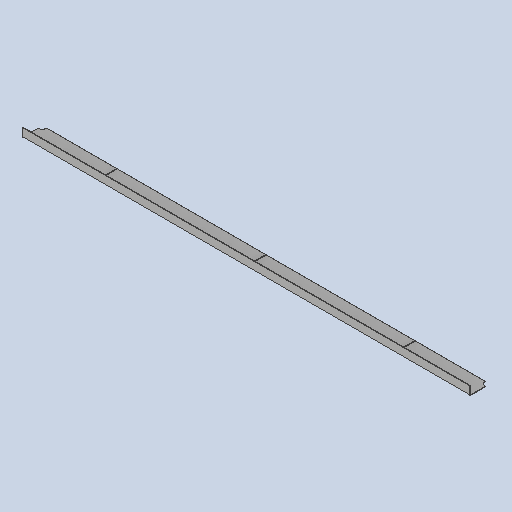
# Autodesk Inventor part: МОО 052 стрингер спина 21
Saved by Autodesk Inventor 2024.2 (Build 282272000, 272)
## iProperties
Created: 2024-04-28
Part Number: МОО 052 стрингер спина 21
Material: Stainless Steel
Document SubType Name: Sheet Metal
Designer: pokla
Density: 8 g/cm^3
Sheet Metal Rule: AISI304 2mm Die16
Appearance: Default
Flat Pattern Width: 9.3976 cm
Flat Pattern Length: 150 cm
Flat Pattern Area: 1409.64 cm^2
Sheet Metal Width: 93,976 mm
Sheet Metal Length: 1500,000 mm
Sheet Metal Area: 140964,031 mm^2
Author: admin
Autodesk Inventor part; units mm, degrees
ref_plane "YZ Plane" through (0, 0, 0) normal (1, 0, 0) x (0, 1, 0)
ref_plane "XZ Plane" through (0, 0, 0) normal (0, 1, 0) x (-1, 0, 0)
ref_plane "XY Plane" through (0, 0, 0) normal (0, 0, 1) x (1, 0, 0)
sketch "Sketch1" plane through (0, 0, 0) normal (0, 0, 1) x (1, 0, 0)
  line L0 (-750, 67.4521) -> (750, 67.4521)
  line L1 (750, 67.4521) -> (750, 0)
  line L2 (750, 0) -> (-750, 0)
  line L3 (-750, 0) -> (-750, 67.4521)
  point P0 (0, 0)
  point P1 (0, 0)
  dimension "d0" = 1500
  dimension "d1" = 67.4521
  measures "d0" distance of L1.end L2.end
  measures "d1" distance of L0.end L1.end
extrude "Plate1" add sketch "Sketch1" along normal blind 2
sketch "Sketch2" plane through (750, 2, 0) normal (0, -1, 0) x (1, 0, 0)
  line L0 (-1500, 0) -> (0, 0)
  line L1 (0, 0) -> (0, 30)
  line L2 (0, 30) -> (-1500, 30)
  line L3 (-1500, 30) -> (-1500, 0)
  constraints: 6 end point, 1 horizontal, 1 perpendicular, 1 vertical
edge flange "Flange1" height 30 angle 90 thickness 2 bend radius 2 thickness toward (0, -1, 0) relief tear relief width 2 relief depth 1 edges at (0, 0, 2) wall of the first edge with corners at (-750, 2, 0) (750, 2, 0) (750, 2, 30) (-750, 2, 30)
bend "Bend1"
corner "Corner1"
sketch "Sketch5" plane through (0, 0, 0) normal (0, 0, -1) x (-1, 0, 0)
  line L0 (750, 67.4521) -> (-750, 67.4521) projected
  line L1 (499, 67.4521) -> (499, 29)
  line L2 (499, 29) -> (501, 29)
  line L3 (501, 29) -> (501, 67.4521)
  line L4 (750, 0) -> (-750, 0) projected
  point P0 (0, 0)
  point P1 (500, 29)
  dimension "d18" = 2
  dimension "d20" = 29
  dimension "d27" = 250
  constraints: 6 end point, 2 perpendicular, 2 point on line, 1 midpoint, 1 vertical
  measures "d18" distance between parallel lines of L3 L1
  measures "d20" distance between parallel lines of L4 L2
  measures "d27" horizontal distance of point (500, 29) L0.start
extrude "Extrusion1" cut sketch "Sketch5" against normal through all
pattern_linear "Rectangular Pattern1" count 3 spacing 500 along (1, 0, 0) of "Extrusion1"
sketch "Sketch6" plane through (0, 0, 0) normal (0, 0, -1) x (-1, 0, 0)
  line L0 (-750, 67.4521) -> (-750, 4) projected
  circle A0 centre (-750, 67.4521) radius 15
  line L1 (-750, 67.4521) -> (-501, 67.4521) projected
  point P0 (0, 0)
  point P1 (-735, 67.4521)
  point P2 (-750, 52.4521)
  dimension "d24" = 30
  constraints: 1 centre point
  measures "d24" diameter of A0
extrude "Extrusion2" cut sketch "Sketch6" against normal through all contours L1 A0 L0 picked at (-740.1254, 66.3395)
mirror "Mirror1" about plane through (0, 0, 0) normal (1, 0, 0) of "Extrusion2"
equation "\"d1\" = Стрингер_2"
equation "\"d18\" = Thickness"
equation "\"d2\" = Thickness"
equation "\"d3\" = BendReliefWidth"
equation "\"d4\" = BendReliefDepth"
equation "\"d5\" = MinimumRemnant"
equation "\"d6\" = TransitionRadius"
equation "\"d9\" = BendRadius"
equation "\"d10\" = CornerReliefSize"
equation "\"d11\" = GapSize"
equation "\"d12\" = JacobiRadiusSize"
equation "\"BendRadius\" = Thickness"
equation "\"BendReliefWidth\" = Thickness"
equation "\"BendReliefDepth\" = 0.5 * Thickness"
equation "\"CornerReliefSize\" = 4 * Thickness"
equation "\"MinimumRemnant\" = 2 * Thickness"
equation "\"TransitionRadius\" = BendRadius"
equation "\"JacobiRadiusSize\" = BendRadius"
equation "\"GapSize\" = Thickness"
equation "\"qqqqqq\" = 67.35706"
equation "\"Стрингер_2\" = 67.452127"
equation "\"Thickness\" = 2"
body "Solid1"
